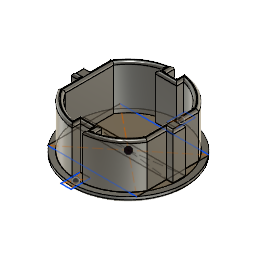
SchukoDustprotector (Autodesk Fusion 360 design; units mm, degrees)
Autodesk Fusion 360 part; units mm, degrees
note: some values were not read from the file. Chosen so that the rebuilt part matches the saved one: which face or edge a step refers to. Set by a fixed rule: which sketch regions a step uses.
sketch "Sketch1" plane through (0, 0, 0) normal (0, 0, 1) x (1, 0, 0)
  circle A0 centre (0, 0) radius 18.5
  line L0 (16, -13) -> (-16, -13)
  line L1 (-16, -13) -> (-16, 13)
  line L2 (-16, 13) -> (16, 13)
  line L3 (16, 13) -> (16, -13)
  line L4 (16, -13) -> (-16, 13) construction
  line L5 (-16, -13) -> (16, 13) construction
  line L6 (18.25, -2.25) -> (-18.25, -2.25)
  line L7 (-18.25, -2.25) -> (-18.25, 2.25)
  line L8 (-18.25, 2.25) -> (18.25, 2.25)
  line L9 (18.25, 2.25) -> (18.25, -2.25)
  line L10 (18.25, -2.25) -> (-18.25, 2.25) construction
  line L11 (-18.25, -2.25) -> (18.25, 2.25) construction
  line L12 (1.85, 22.1922) -> (-1.85, 22.1922)
  line L13 (-1.85, 22.1922) -> (-1.85, 15.5)
  line L14 (-1.85, 15.5) -> (1.85, 15.5)
  line L15 (1.85, 15.5) -> (1.85, 22.1922)
  line L16 (1.85, 22.1922) -> (-1.85, 15.5) construction
  line L17 (-1.85, 22.1922) -> (1.85, 15.5) construction
  line L18 (1.8657, -22.4776) -> (-1.8343, -22.4776)
  line L19 (-1.8343, -22.4776) -> (-1.8343, -15.5)
  line L20 (-1.8343, -15.5) -> (1.8657, -15.5)
  line L21 (1.8657, -15.5) -> (1.8657, -22.4776)
  line L22 (1.8657, -22.4776) -> (-1.8343, -15.5) construction
  line L23 (-1.8343, -22.4776) -> (1.8657, -15.5) construction
  point P0 (0, 18.8461)
  point P1 (0.0157, -18.9888)
  dimension "d1" = 37
  dimension "d2" = 32
  dimension "d4" = 36.5
  dimension "d5" = 4.5
  dimension "d6" = 3.7
  dimension "d9" = 3.7
  dimension "d20" = 15.5
  dimension "d21" = 15.5
  measures "d1" diameter of A0
  measures "d2" distance of L1.end L2.end
  measures "d4" distance of L7.end L8.end
  measures "d5" distance of L6.end L7.end
  measures "d6" distance of L13.end L14.end
  measures "d9" distance of L19.end L20.end
  measures "d20" distance of A0.centre L14
  measures "d21" distance of A0.centre L20
extrude "Extrude1" add sketch "Sketch1" along normal blind 16 contours A0 L1 L2 L3 L8 | A0 L0 L1 L3 L6 | A0 L2 L13 L14 L15 | L3 L6 L8 L9 | L1 L3 L6 L8 | A0 L0 L19 L20 L21 | L1 L6 L7 L8 makes body 1
sketch "Sketch2" plane through (0, 0, 0) normal (0, 0, 1) x (1, 0, 0)
  circle A0 centre (0, 0) radius 20.5
  dimension "d19" = 41
  measures "d19" diameter of A0
extrude "Extrude2" add sketch "Sketch2" against normal blind 2 bodies 1
fillet "Fillet1" radius 1 1 edges at (-20.5, 0, -2) on bodies 1
shell "Shell1" thickness 2 removed faces 1 at (-6.5614, 0.75, 16) on bodies 1
move_face "OffsetFaces1" offset 2.25 1 faces at (16.25, 0.0833, 5.3333) on bodies 1
move_face "OffsetFaces2" offset 2.25 1 faces at (-16.25, -0.0833, 5.3333) on bodies 1
copy_body "Body->Comp1" bodies 1 removing the originals makes body 2 in component "PODustCover"
fillet "Fillet1'" radius 0.85 32 edges at (-14, 0, 16) (-9.6383, -13.3923, 16) (-3.8343, -14.7742, 16) (0.0157, -13.5, 16) (3.8657, -14.7704, 16) (9.6514, -13.3828, 16) (14, 0, 16) (9.6449, 13.3876, 16) (3.85, 14.7723, 16) (0, 13.5, 16) (-3.85, 14.7723, 16) (-9.6449, 13.3876, 16) (16, 5.7685, 16) (17.125, 2.25, 16) (18.25, 0, 16) (17.125, -2.25, 16) (16, -5.7685, 16) (10.0291, -15.5456, 16) (1.8657, -16.9528, 16) (0.0157, -15.5, 16) (-1.8343, -16.9544, 16) (-10.0159, -15.5542, 16) (-16, -5.7685, 16) (-17.125, -2.25, 16) (-18.25, 0, 16) (-17.125, 2.25, 16) (-16, 5.7685, 16) (-10.0225, 15.5499, 16) (-1.85, 16.9536, 16) (0, 15.5, 16) (1.85, 16.9536, 16) (10.0225, 15.5499, 16) on bodies 2 in component "PODustCover"
component "PODustCover" placed x (1, 0, 0) y (0, 1, 0) z (0, 0, 1) at (0, 0, 0)
